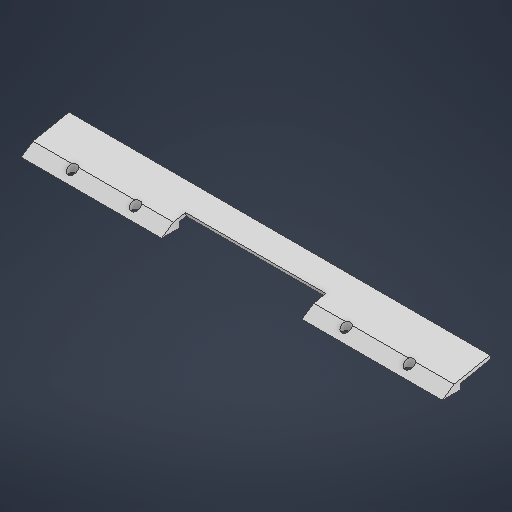
# Autodesk Inventor part: przod
Saved by Autodesk Inventor 2026.2 (Build 302298010, 298A)
## iProperties
Created: 2026-05-13
Part Number: przod
Material: Generic
Document SubType Name: Modeling
Designer: karol
Density: 1 g/cm^3
Appearance: Default
Author: karol
Autodesk Inventor part; units mm, degrees
ref_plane "YZ Plane" through (0, 0, 0) normal (1, 0, 0) x (0, 1, 0)
ref_plane "XZ Plane" through (0, 0, 0) normal (0, 1, 0) x (-1, 0, 0)
ref_plane "XY Plane" through (0, 0, 0) normal (0, 0, 1) x (1, 0, 0)
sketch "Sketch1" plane through (0, 0, 0) normal (1, 0, 0) x (0, 1, 0)
  line L0 (0, 0) -> (0, -6.5)
  line L1 (0, -6.5) -> (2, -6.5)
  line L2 (2, -6.5) -> (4.16, -17.286)
  line L3 (0, 0) -> (2, 0)
  line L4 (2, 0) -> (5.4115, -17.0354)
  line L5 (5.4115, -17.0354) -> (4.16, -17.286)
  dimension "d0" = 6.5
  dimension "d1" = 2
  dimension "d2" = 10.786
  dimension "d3" = 2.16
  constraints: 12 end point, 2 perpendicular, 1 horizontal, 1 vertical
  measures "d0" distance of L0.start L0.end
  measures "d1" distance of L0.end L1.end
  measures "d2" vertical distance of L2.end L1.end
  measures "d3" horizontal distance of L2.end L1.end
extrude "Extrusion1" add sketch "Sketch1" along normal blind 50
sketch "Sketch2" plane through (50, 0, 0) normal (1, 0, 0) x (0, 0, -1)
  line L0 (0, 0) -> (6.5, 0) projected
  line L1 (6.5, 0) -> (6.5, 2) projected
  line L2 (6.5, 2) -> (17.286, 4.16) projected
  line L3 (17.286, 4.16) -> (17.0354, 5.4115) projected
  line L4 (17.0354, 5.4115) -> (0, 2) projected
  line L5 (0, 2) -> (0, 0) projected
  line L6 (8.7683, 2.4543) -> (8.5177, 3.7057)
  constraints: 2 end point, 1 midpoint, 1 point on line
extrude "Extrusion2" add sketch "Sketch2" along normal blind 50 contours L4 L3 L2 L6
sketch "Sketch3" plane through (100, 0, 0) normal (1, 0, 0) x (0, 0, -1)
  line L0 (8.7683, 2.4543) -> (8.5177, 3.7057) projected
  line L1 (8.5177, 3.7057) -> (0, 2) projected
  line L2 (0, 2) -> (0, 0) projected
  line L3 (0, 0) -> (6.5, 0) projected
  line L4 (6.5, 0) -> (6.5, 2) projected
  line L5 (6.5, 2) -> (8.7683, 2.4543) projected
  line L6 (17.0354, 5.4115) -> (8.5177, 3.7057) projected
  line L7 (8.5177, 3.7057) -> (8.7683, 2.4543) projected
  line L8 (8.7683, 2.4543) -> (17.286, 4.16) projected
  line L9 (17.286, 4.16) -> (17.0354, 5.4115) projected
extrude "Extrusion3" add sketch "Sketch3" along normal blind 50
sketch "Sketch4" plane through (100, 0, -6.5) normal (0, -1, 0) x (1, 0, 0)
  circle A0 centre (-85, 3.25) radius 1.55
  circle A1 centre (-62.5, 3.25) radius 1.55
  line L0 (-100, 6.5) -> (-100, 0) projected
  line L1 (-100, 6.5) -> (-50, 6.5) projected
  circle A2 centre (35, 3.25) radius 1.55
  circle A3 centre (12.5, 3.25) radius 1.55
  line L2 (0, 6.5) -> (50, 6.5) projected
  line L3 (50, 6.5) -> (50, 0) projected
  point P0 (-100, 3.25)
  dimension "d10" = 37.5
  dimension "d11" = 15
  dimension "d12" = 3.25
  dimension "d13" = 3.1
  dimension "d14" = 3.25
  dimension "d15" = 3.1
  dimension "d16" = 3.1
  dimension "d17" = 3.1
  dimension "d18" = 3.25
  dimension "d19" = 3.25
  dimension "d20" = 15
  dimension "d21" = 37.5
  constraints: 4 centre point, 1 midpoint
  measures "d10" distance of point (-100, 3.25) A1.centre
  measures "d11" distance from line of A0.centre L0
  measures "d12" distance from line of L1 A1.centre
  measures "d13" diameter of A1
  measures "d14" distance from line of L1 A0.centre
  measures "d15" diameter of A0
  measures "d16" diameter of A2
  measures "d17" diameter of A3
  measures "d18" distance from line of L2 A3.centre
  measures "d19" distance from line of L2 A2.centre
  measures "d20" distance from line of L3 A2.centre
  measures "d21" distance from line of A3.centre L3
extrude "Extrusion4" cut sketch "Sketch4" against normal blind 3
sketch "Sketch5" plane through (150, 0, 0) normal (1, 0, 0) x (0, 0, -1)
  line L0 (0, 0) -> (13.9221, 9.3906)
  line L1 (0, 0) -> (16.7931, 0) construction
  line L2 (0, 0) -> (4.2172, 2.8445)
  line L3 (1.7, 2.3404) -> (4.8, 2.9612) projected
  line L4 (17.0354, 5.4115) -> (0, 2) projected
  line L5 (0, 2) -> (4.2172, 2.8445)
  line L6 (0, 2) -> (0, 0)
  dimension "d24" = 34
  constraints: 10 end point, 2 point on line, 1 collinear, 1 equal length, 1 horizontal, 1 perpendicular
  measures "d24" angle of L1 L0
extrude "Extrusion5" cut sketch "Sketch5" against normal blind 150
body "Solid1"
